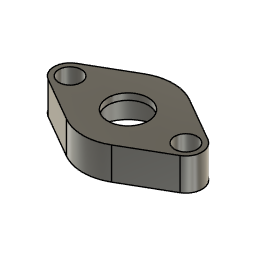
magnet_mount (Autodesk Fusion 360 design; units mm, degrees)
Autodesk Fusion 360 part; units mm, degrees
note: some values were not read from the file. Set by a fixed rule: which sketch regions a step uses.
sketch "Sketch1" plane through (0, 0, 0) normal (0, 0, 1) x (1, 0, 0)
  circle A0 centre (0, 0) radius 5.15
  circle A1 centre (0, 0) radius 7
  circle A2 centre (9, 0) radius 2.5
  circle A3 centre (-9, 0) radius 2.5
  circle A4 centre (-9, 0) radius 1.75
  circle A5 centre (9, 0) radius 1.75
  line L0 (-10.25, 2.1651) -> (-3.5, 6.0622)
  line L1 (-9, 0) -> (9, 0)
  line L2 (-10.25, -2.1651) -> (-3.5, -6.0622)
  line L3 (0, 12) -> (0, 15)
  line L4 (10.25, 2.1651) -> (3.5, 6.0622)
  line L5 (10.25, -2.1651) -> (3.5, -6.0622)
  dimension "d1" = 10.3
  dimension "d2" = 14
  dimension "d3" = 5
  dimension "d4" = 5
  dimension "d5" = 9
  dimension "d6" = 9
  dimension "d7" = 3.5
  dimension "d8" = 3.5
  constraint coincident A0.centre A1.centre
  constraint concentric A0 A1
  constraint concentric A3 A4
  constraint concentric A2 A5
  constraint tangent A1 L0
  constraint coincident A3.centre A4.centre
  constraint coincident A2.centre A5.centre
  constraint horizontal L1
  constraint tangent A3 L0
  constraint tangent A1 L2
  constraint tangent A3 L2
  constraint coincident A1 L0.end
  constraint coincident A1 L2.end
  constraint coincident A3 L2.start
  constraint coincident A3 L0.start
  constraint vertical L3
  constraint symmetric L0.end L3 L4.end
  constraint symmetric L2.end L3 L5.end
  constraint symmetric L2.start L3 L5.start
  constraint symmetric L0.start L3 L4.start
  constraint coincident A1 L5.end
  measures "d1" diameter of A0
  measures "d2" diameter of A1
  measures "d3" diameter of A2
  measures "d4" diameter of A3
  measures "d5" distance of A0.centre A3.centre
  measures "d6" distance of A0.centre A2.centre
  measures "d7" diameter of A4
  measures "d8" diameter of A5
extrude "Extrude1" add sketch "Sketch1" along normal blind 5 contours A0 A1 A2 A3 L1 | A0 A1 A2 A3 L1 | A1 A2 L1 | A1 A2 L1 | A1 A3 L1 | A1 A3 L1 | A1 A2 | A1 A2 L4 | A1 A2 L5 | A1 A3 L0 | A1 A3 | A1 A3 L2
sketch "Sketch2" plane through (0, 0, 5) normal (0, 0, 1) x (-1, 0, 0)
  circle A0 centre (-9, 0) radius 1.75
  circle A1 centre (0, 0) radius 5.15
  circle A2 centre (9, 0) radius 1.75
  line L0 (-10.25, -2.1651) -> (-3.5, -6.0622)
  arc A3 (-3.5, -6.0622) -> (3.5, -6.0622) centre (0, 0) ccw
  line L1 (3.5, -6.0622) -> (10.25, -2.1651)
  arc A4 (10.25, -2.1651) -> (10.25, 2.1651) centre (9, 0) ccw
  line L2 (10.25, 2.1651) -> (3.5, 6.0622)
  arc A5 (3.5, 6.0622) -> (-3.5, 6.0622) centre (0, 0) ccw
  line L3 (-3.5, 6.0622) -> (-10.25, 2.1651)
  arc A6 (-10.25, 2.1651) -> (-10.25, -2.1651) centre (-9, 0) ccw
  circle A7 centre (0, 0) radius 3.15
  dimension "d11" = -2
extrude "Extrude2" add sketch "Sketch2" against normal blind 1 contours A1
